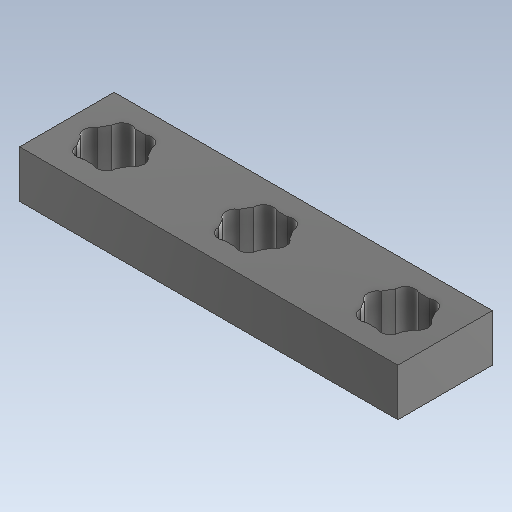
# Autodesk Inventor part: Trunk_abdomen_spacer
Saved by Autodesk Inventor 2020.4 (Build 244396000, 396)
## iProperties
Created: 2021-09-11
Part Number: Trunk_abdomen_spacer
Material: アセタール樹脂、黒
Document SubType Name: Modeling
Designer: Masato
Density: 1.425 g/cm^3
Appearance: 滑らか - 黒
Mass: 2.26034 g
Surface Area: 14.3023 cm^2
Volume: 1.5862 cm^3
Description: POM T5
Author: Masato Kubotera
Autodesk Inventor part; units mm, degrees
ref_plane "YZ Plane" through (0, 0, 0) normal (1, 0, 0) x (0, 1, 0)
ref_plane "XZ Plane" through (0, 0, 0) normal (0, 1, 0) x (-1, 0, 0)
ref_plane "XY Plane" through (0, 0, 0) normal (0, 0, 1) x (1, 0, 0)
derived "Trunk_vertical_frame_03.ipt"
sketch "スケッチ1" plane through (0, 0, 0) normal (0, 0, 1) x (1, 0, 0)
  circle A0 centre (0, 0) radius 11
  line L0 (1, 13.5) -> (28, 13.5) construction
  line L1 (28, 13.5) -> (28, -13.5) construction
  line L2 (28, -13.5) -> (1, -13.5) construction
  line L3 (1, -13.5) -> (1, 13.5) construction
  line L4 (1, 13.5) -> (28, -13.5) construction
  line L5 (28, 13.5) -> (1, -13.5) construction
  line L6 (-12, 16) -> (39.5, 16) construction
  line L7 (39.5, 16) -> (39.5, -16) construction
  line L8 (39.5, -16) -> (-12, -16) construction
  line L9 (-12, -16) -> (-12, 16) construction
  line L10 (-12, 16) -> (39.5, -16) construction
  line L11 (39.5, 16) -> (-12, -16) construction
  circle A1 centre (1, 13.5) radius 1.35
  arc A2 (0, 16) -> (-12, 10.583) centre (0, 0) ccw construction
  line L12 (-12, 0) -> (39.5, 0)
  circle A3 centre (28, 13.5) radius 1.35
  arc A4 (-12, -10.583) -> (0, -16) centre (0, 0) ccw construction
  circle A5 centre (28, -13.5) radius 1.35
  circle A6 centre (1, -13.5) radius 1.35
  arc A7 (0, 16.01) -> (-12.01, 10.5868) centre (0, 0) ccw
  line L13 (0, 16.01) -> (39.51, 16.01)
  line L14 (39.51, 16.01) -> (39.51, 13.26)
  line L15 (-12.01, 10.5868) -> (-12.01, 0)
  arc A8 (-11.4729, 11.1666) -> (-12.01, 9.8444) centre (-11.0278, 10.2156) ccw
  line L16 (-12.01, 10.5868) -> (-11.0278, 10.2156) construction
  arc A9 (39.51, 14.5251) -> (38.0251, 16.01) centre (38.7675, 15.2675) ccw
  line L17 (38.7675, 15.2675) -> (39.51, 16.01) construction
  arc A10 (38.0251, -16.01) -> (39.51, -14.5251) centre (38.7675, -15.2675) ccw
  line L18 (-12.01, -10.5868) -> (-12.01, 0)
  arc A11 (-12.01, -9.8444) -> (-11.4729, -11.1666) centre (-11.0278, -10.2156) ccw
  arc A12 (-12.01, -10.5868) -> (0, -16.01) centre (0, 0) ccw
  line L19 (0, -16.01) -> (39.51, -16.01)
  line L20 (39.51, 13.26) -> (42.01, 13.26)
  line L21 (42.01, 13.26) -> (42.01, -1.76)
  line L22 (42.01, -1.76) -> (39.51, -1.76)
  line L23 (39.51, -1.76) -> (39.51, -14.5251)
  line L24 (39.5, 13.25) -> (42, 13.25) construction
  line L25 (42, 13.25) -> (42, -1.75) construction
  line L26 (42, -1.75) -> (39.5, -1.75) construction
  line L27 (42, 5.75) -> (39.5, 5.75) construction
  arc A13 (42.01, 11.7751) -> (40.5251, 13.26) centre (41.2675, 12.5175) ccw
  line L28 (41.2675, 12.5175) -> (42.01, 13.26) construction
  arc A14 (40.5251, -1.76) -> (42.01, -0.2751) centre (41.2675, -1.0175) ccw
  circle A15 centre (-15.5, 19) radius 1.55
  line L29 (-18, 22) -> (-13, 22) construction
  line L30 (-13, 22) -> (-13, -10.5) construction
  line L31 (-13, -10.5) -> (-18, -10.5) construction
  line L32 (-18, -10.5) -> (-18, 22) construction
  line L33 (-18, 22) -> (-13, -10.5) construction
  line L34 (-13, 22) -> (-18, -10.5) construction
  line L35 (-18, 5.75) -> (-13, 5.75) construction
  line L36 (-15.5, 22) -> (-15.5, -10.5) construction
  line L37 (-18, 13.25) -> (-15.5, 13.25) construction
  line L38 (-15.5, 13.25) -> (-15.5, -1.75) construction
  line L39 (-15.5, -1.75) -> (-18, -1.75) construction
  line L40 (-18, 13.25) -> (-15.5, -1.75) construction
  line L41 (-15.5, 13.25) -> (-18, -1.75) construction
  line L42 (-15.49, -1.76) -> (-18.01, -1.76)
  line L43 (-18.01, -1.76) -> (-18.01, 13.26)
  line L44 (-18.01, 13.26) -> (-15.49, 13.26)
  line L45 (-15.49, 13.26) -> (-15.49, -1.76)
  line L46 (-15.49, -1.76) -> (-18.01, 13.26) construction
  line L47 (-18.01, -1.76) -> (-15.49, 13.26) construction
  line L48 (-16.75, 13.26) -> (-16.75, -1.76) construction
  arc A16 (-18.01, 13.26) -> (-18.01, 11.16) centre (-18.01, 12.21) ccw
  arc A17 (-15.49, 11.16) -> (-15.49, 13.26) centre (-15.49, 12.21) ccw
  arc A18 (-18.01, 0.34) -> (-18.01, -1.76) centre (-18.01, -0.71) ccw
  arc A19 (-15.49, -1.76) -> (-15.49, 0.34) centre (-15.49, -0.71) ccw
  circle A20 centre (-15.5, -7.5) radius 1.55
  line L49 (14.5, 16) -> (14.5, -16) construction
  circle A21 centre (42, 19) radius 1.55
  line L50 (39.5, 22) -> (44.5, 22) construction
  line L51 (44.5, 22) -> (44.5, -10.5) construction
  line L52 (44.5, -10.5) -> (39.5, -10.5) construction
  line L53 (39.5, 22) -> (44.5, -10.5) construction
  line L54 (44.5, 22) -> (39.5, -10.5) construction
  line L55 (42, 22) -> (42, -10.5) construction
  circle A22 centre (42, -7.5) radius 1.55
  line L56 (-12, -18.25) -> (27, -18.25) construction
  line L57 (27, -18.25) -> (27, -23.25) construction
  line L58 (27, -23.25) -> (-12, -23.25) construction
  line L59 (-12, -23.25) -> (-12, -18.25) construction
  line L60 (-12, -18.25) -> (27, -23.25) construction
  line L61 (27, -18.25) -> (-12, -23.25) construction
  line L62 (-3, -20.75) -> (18, -20.75) construction
  line L63 (18, -20.75) -> (18, -18.25) construction
  line L64 (-3, -18.25) -> (-3, -20.75) construction
  line L65 (-3, -20.75) -> (18, -18.25) construction
  line L66 (18, -20.75) -> (-3, -18.25) construction
  line L67 (-12, -20.75) -> (27, -20.75) construction
  line L68 (7.5, -18.25) -> (7.5, -23.25) construction
  line L69 (-3.01, -18.24) -> (18.01, -18.24)
  line L70 (18.01, -18.24) -> (18.01, -20.76)
  line L71 (18.01, -20.76) -> (-3.01, -20.76)
  line L72 (-3.01, -20.76) -> (-3.01, -18.24)
  line L73 (-3.01, -18.24) -> (18.01, -20.76) construction
  line L74 (18.01, -18.24) -> (-3.01, -20.76) construction
  circle A23 centre (-8, -20.75) radius 1.55
  circle A24 centre (23, -20.75) radius 1.55
  arc A25 (-0.91, -18.24) -> (-3.01, -18.24) centre (-1.96, -18.24) ccw
  arc A26 (18.01, -18.24) -> (15.91, -18.24) centre (16.96, -18.24) ccw
  line L75 (-3.01, -19.5) -> (18.01, -19.5) construction
  arc A27 (-3.01, -20.76) -> (-0.91, -20.76) centre (-1.96, -20.76) ccw
  arc A28 (15.91, -20.76) -> (18.01, -20.76) centre (16.96, -20.76) ccw
  circle A29 centre (-8, 20.75) radius 1.55
  line L76 (18.01, 20.76) -> (-3.01, 20.76)
  line L77 (-3.01, 19.5) -> (18.01, 19.5) construction
  line L78 (-3, 18.25) -> (-3, 20.75) construction
  line L79 (18, 20.75) -> (-3, 18.25) construction
  line L80 (-3, 20.75) -> (18, 18.25) construction
  line L81 (-3.01, 20.76) -> (-3.01, 18.24)
  line L82 (-3.01, 18.24) -> (18.01, 20.76) construction
  line L83 (-3.01, 18.24) -> (18.01, 18.24)
  arc A30 (-3.01, 18.24) -> (-0.91, 18.24) centre (-1.96, 18.24) ccw
  line L84 (18.01, 18.24) -> (-3.01, 20.76) construction
  line L85 (-12, 23.25) -> (-12, 18.25) construction
  arc A31 (-0.91, 20.76) -> (-3.01, 20.76) centre (-1.96, 20.76) ccw
  line L86 (7.5, 18.25) -> (7.5, 23.25) construction
  line L87 (-3, 20.75) -> (18, 20.75) construction
  line L88 (-12, 20.75) -> (27, 20.75) construction
  line L89 (27, 23.25) -> (-12, 23.25) construction
  line L90 (-12, 18.25) -> (27, 18.25) construction
  line L91 (-12, 18.25) -> (27, 23.25) construction
  line L92 (27, 18.25) -> (-12, 23.25) construction
  line L93 (27, 18.25) -> (27, 23.25) construction
  arc A32 (15.91, 18.24) -> (18.01, 18.24) centre (16.96, 18.24) ccw
  circle A33 centre (23, 20.75) radius 1.55
  line L94 (18, 20.75) -> (18, 18.25) construction
  line L95 (18.01, 18.24) -> (18.01, 20.76)
  arc A34 (18.01, 20.76) -> (15.91, 20.76) centre (16.96, 20.76) ccw
  line L96 (-18, 28.25) -> (44.5, 28.25)
  line L97 (-18, 28.25) -> (-23, 22)
  line L98 (44.5, 28.25) -> (47.5, 22)
  line L99 (-23, 22) -> (-23, -2.875)
  line L100 (47.5, 22) -> (47.5, -18.25)
  line L101 (47.5, -18.25) -> (37, -33.25)
  line L102 (-23, -2.875) -> (-33.5, -16)
  line L103 (-33.5, -16) -> (-33.5, -87)
  line L104 (37, -33.25) -> (37, -70.3333)
  line L105 (37, -70.3333) -> (23, -96)
  line L106 (23, -96) -> (-17, -96)
  line L107 (-17, -96) -> (-33.5, -87)
  circle A35 centre (-12, -91) radius 1.55
  circle A36 centre (3, -91) radius 1.55
  line L108 (-17, -96) -> (-17, -86)
  line L109 (-17, -86) -> (23, -86)
  line L110 (23, -86) -> (23, -96)
  line L111 (-17, -91) -> (23, -91) construction
  line L112 (3, -86) -> (3, -96) construction
  circle A37 centre (18, -91) radius 1.55
  circle A38 centre (-13.5, -56.75) radius 1.55
  line L113 (-23.5, -60.75) -> (27, -60.75)
  line L114 (27, -60.75) -> (27, -76)
  line L115 (27, -76) -> (-23.5, -76)
  line L116 (-23.5, -76) -> (-23.5, -60.75)
  line L117 (-23.5, -33.25) -> (27, -33.25)
  line L118 (27, -33.25) -> (27, -52.75)
  line L119 (27, -52.75) -> (-23.5, -52.75)
  line L120 (-23.5, -52.75) -> (-23.5, -33.25)
  circle A39 centre (-13.5, -56.75) radius 4 construction
  arc A40 (-11.4565, -93.76) -> (-9.8815, -92.8507) centre (-10.9315, -92.8507) ccw
  line L121 (-9.338, -91.9093) -> (-9.8815, -92.8507)
  arc A41 (-9.338, -91.9093) -> (-9.338, -90.0907) centre (-9.863, -91) ccw
  line L122 (-9.8815, -89.1493) -> (-9.338, -90.0907)
  arc A42 (-9.8815, -89.1493) -> (-11.4565, -88.24) centre (-10.9315, -89.1493) ccw
  line L123 (-12.5435, -88.24) -> (-11.4565, -88.24)
  arc A43 (-12.5435, -88.24) -> (-14.1185, -89.1493) centre (-13.0685, -89.1493) ccw
  line L124 (-14.662, -90.0907) -> (-14.1185, -89.1493)
  arc A44 (-14.662, -90.0907) -> (-14.662, -91.9093) centre (-14.137, -91) ccw
  line L125 (-14.1185, -92.8507) -> (-14.662, -91.9093)
  arc A45 (-14.1185, -92.8507) -> (-12.5435, -93.76) centre (-13.0685, -92.8507) ccw
  line L126 (-11.4565, -93.76) -> (-12.5435, -93.76)
  arc A46 (5.662, -91.9093) -> (5.662, -90.0907) centre (5.137, -91) ccw
  line L127 (5.1185, -89.1493) -> (5.662, -90.0907)
  line L128 (5.662, -91.9093) -> (5.1185, -92.8507)
  arc A47 (3.5435, -93.76) -> (5.1185, -92.8507) centre (4.0685, -92.8507) ccw
  arc A48 (5.1185, -89.1493) -> (3.5435, -88.24) centre (4.0685, -89.1493) ccw
  line L129 (2.4565, -88.24) -> (3.5435, -88.24)
  arc A49 (2.4565, -88.24) -> (0.8815, -89.1493) centre (1.9315, -89.1493) ccw
  line L130 (0.338, -90.0907) -> (0.8815, -89.1493)
  arc A50 (0.338, -90.0907) -> (0.338, -91.9093) centre (0.863, -91) ccw
  line L131 (0.8815, -92.8507) -> (0.338, -91.9093)
  arc A51 (0.8815, -92.8507) -> (2.4565, -93.76) centre (1.9315, -92.8507) ccw
  line L132 (3.5435, -93.76) -> (2.4565, -93.76)
  arc A52 (20.662, -91.9093) -> (20.662, -90.0907) centre (20.137, -91) ccw
  line L133 (20.1185, -89.1493) -> (20.662, -90.0907)
  line L134 (20.662, -91.9093) -> (20.1185, -92.8507)
  arc A53 (18.5435, -93.76) -> (20.1185, -92.8507) centre (19.0685, -92.8507) ccw
  arc A54 (20.1185, -89.1493) -> (18.5435, -88.24) centre (19.0685, -89.1493) ccw
  line L135 (17.4565, -88.24) -> (18.5435, -88.24)
  arc A55 (17.4565, -88.24) -> (15.8815, -89.1493) centre (16.9315, -89.1493) ccw
  line L136 (15.338, -90.0907) -> (15.8815, -89.1493)
  arc A56 (15.338, -90.0907) -> (15.338, -91.9093) centre (15.863, -91) ccw
  line L137 (15.8815, -92.8507) -> (15.338, -91.9093)
  arc A57 (15.8815, -92.8507) -> (17.4565, -93.76) centre (16.9315, -92.8507) ccw
  line L138 (18.5435, -93.76) -> (17.4565, -93.76)
  point P0 (14.5, 0)
  point P1 (-15.5, 5.75)
  point P2 (-16.75, 5.75)
  point P3 (14.5, 0)
  point P4 (42, 5.75)
  point P5 (42, 5.75)
  point P6 (7.5, -20.75)
  point P7 (7.5, -19.5)
  point P8 (7.5, -19.5)
  point P9 (7.5, -19.5)
  point P10 (7.5, -19.5)
  point P11 (7.5, 20.75)
  point P12 (7.5, 19.5)
  point P13 (7.5, 19.5)
  point P14 (7.5, 19.5)
  point P15 (7.5, 19.5)
  point P16 (-10.4065, -93.76)
  point P17 (-8.813, -91)
  point P18 (-10.4065, -88.24)
  point P19 (-13.5935, -88.24)
  point P20 (-13.5935, -88.24)
  point P21 (-15.187, -91)
  point P22 (-13.5935, -93.76)
  point P23 (-15.187, -91)
  point P24 (-8.813, -91)
  point P25 (3, -91)
  point P26 (6.187, -91)
  point P27 (6.187, -91)
  point P28 (4.5935, -88.24)
  point P29 (4.5935, -93.76)
  point P30 (3, -91)
  point P31 (3, -91)
  point P32 (1.4065, -88.24)
  point P33 (1.4065, -88.24)
  point P34 (-0.187, -91)
  point P35 (-0.187, -91)
  point P36 (1.4065, -93.76)
  point P37 (18, -91)
  point P38 (21.187, -91)
  point P39 (21.187, -91)
  point P40 (19.5935, -88.24)
  point P41 (19.5935, -93.76)
  point P42 (18, -91)
  point P43 (18, -91)
  point P44 (16.4065, -88.24)
  point P45 (16.4065, -88.24)
  point P46 (14.813, -91)
  point P47 (14.813, -91)
  point P48 (16.4065, -93.76)
  point P49 (15.8815, -89.1493)
  point P50 (0.8815, -89.1493)
  point P51 (-14.1185, -89.1493)
extrude "押し出し1" add sketch "スケッチ1" along normal blind 5 contours L108 L109 L110 L106
